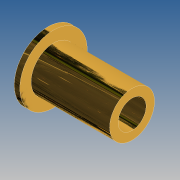
# Autodesk Inventor part: M003
Saved by Autodesk Inventor 2017 (Build 210142000, 142)
## iProperties
Created: 2018-10-12
Part Number: M003
Material: Laiton / Messing
Document SubType Name: Modeling
Designer: Gilles Mottiez
Density: 8.47 g/cm^3
Appearance: Laiton - Satiné
Description: Palier demi-coque de face
Mass: 4.42379 g
Surface Area: 8.12102 cm^2
Volume: 0.52229 cm^3
Author: Gilles Mottiez
Autodesk Inventor part; units mm, degrees
ref_plane "YZ Plane" through (0, 0, 0) normal (1, 0, 0) x (0, 1, 0)
ref_plane "XZ Plane" through (0, 0, 0) normal (0, 1, 0) x (-1, 0, 0)
ref_plane "XY Plane" through (0, 0, 0) normal (0, 0, 1) x (1, 0, 0)
sketch "Sketch1" plane through (0, 0, 0) normal (0, 0, 1) x (1, 0, 0)
  line L0 (0, 0) -> (15, 0) construction
  line L1 (0, 0) -> (0, 15) construction
  line L2 (15, 0) -> (15, 15) construction
  line L3 (0, 6) -> (0, 2.5)
  line L4 (15, 2.5) -> (0, 2.5)
  line L5 (0, 6) -> (1, 6)
  line L6 (1, 6) -> (1, 4)
  line L7 (1, 4) -> (15, 4)
  line L8 (15, 4) -> (15, 2.5)
  dimension "d0" = 15
  dimension "d1" = 15
  dimension "d2" = 15
  dimension "d3" = 5
  dimension "d4" = 8
  dimension "d5" = 12
  dimension "d6" = 1
  constraints: 18 end point, 4 point on line, 3 perpendicular, 2 horizontal, 2 vertical, 1 collinear
  measures "d0" distance of L0.start L1.end
  measures "d1" distance of L0.end L2.end
  measures "d2" distance between parallel lines of L2 L1
  measures "d3" diameter of L4 L0
  measures "d4" diameter of L7 L0
  measures "d5" diameter of L5 L0
  measures "d6" distance of L3.start L5.end
revolve "Révolution1" add sketch "Sketch1" angle 360 about axis through (0, 0, 0) along (1, 0, 0)
